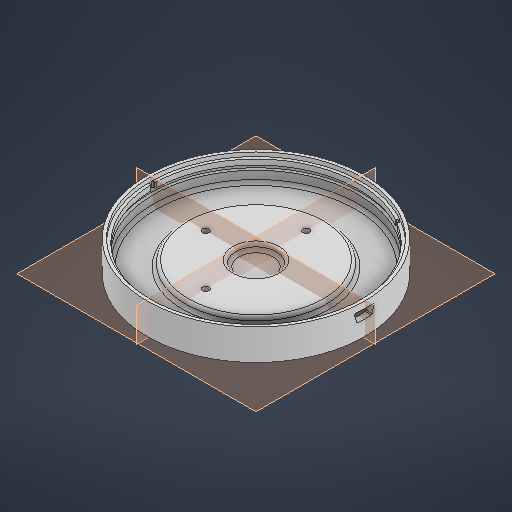
# Autodesk Inventor part: housing
Saved by Autodesk Inventor 2026 (Build 300175050, 175E)
## iProperties
Created: 2025-07-28
Part Number: housing
Material: Generic
Document SubType Name: Modeling
Designer: bruno
Density: 1 g/cm^3
Appearance: Default
Author: bruno
Autodesk Inventor part; units mm, degrees
sketch "Sketch3" plane through (0, 0, 0) normal (0, 1, 0) x (-1, 0, 0)
  circle A0 centre (0, 0) radius 54
  dimension "d4" = 108
  constraints: 1 centre point, 1 coincident
  measures "d4" diameter of A0
extrude "Extrusion2" add sketch "Sketch3" along normal blind 15.3
shell "Shell1" thickness 3 removed faces 1 at (7.7603, 15.3, 10.4365)
ref_plane "Work Plane1" through (54, 0, 0) normal (1, 0, 0) x (0, 1, 0)
sketch "Sketch5" plane through (54, 0, 0) normal (1, 0, 0) x (0, 1, 0)
  line L0 (12, 5) -> (7.5, 3.75)
  line L1 (7.5, 3.75) -> (7.5, -3.75)
  line L2 (7.5, -3.75) -> (12, -5)
  line L3 (12, -5) -> (12, 5)
  line L4 (-2.4, 0) -> (14.4, 0) projected
  line L5 (0, 7) -> (0, -7) projected
  point P0 (0, 0)
  point P1 (12, 0)
  point P2 (7.5, 0)
  dimension "d13" = 4.5
  dimension "d14" = 7.5
  dimension "d16" = 5
  dimension "d17" = 7.5
  constraints: 8 end point, 2 horizontal alignment, 2 midpoint
  measures "d13" distance between parallel lines of L3 L1
  measures "d14" distance between parallel lines of L5 L1
  measures "d16" distance from line of L4 L0.start
  measures "d17" distance of L0.end L1.end
extrude "Extrusion3" cut sketch "Sketch5" against normal blind 6
fillet "Fillet1" radius 0.5 4 edges at (52.3658, 7.5, -3.75) (52.2612, 12, -5) (52.2612, 12, 5) (52.3658, 7.5, 3.75)
sketch "Sketch6" plane through (0, 3, 0) normal (0, 1, 0) x (1, 0, 0)
  circle A0 centre (0, 0) radius 35
  circle A1 centre (0, 0) radius 10
  dimension "d19" = 70
  dimension "d22" = 20
  constraints: 2 centre point, 2 coincident
  measures "d19" diameter of A0
  measures "d22" diameter of A1
extrude "Extrusion5" add sketch "Sketch6" along normal blind 3
sketch "Sketch7" plane through (0, 0, 0) normal (0, -1, 0) x (1, 0, 0)
  circle A0 centre (0, 0) radius 35 projected
  circle A1 centre (0, 0) radius 10 projected
  circle A2 centre (0, 0) radius 54 projected
  circle A3 centre (0, 0) radius 32
  circle A4 centre (0, 0) radius 13
  dimension "d25" = 3
  dimension "d26" = 3
  constraints: 2 centre point
  measures "d25" radial gap between concentric circles of A0 A3
  measures "d26" radial gap between concentric circles of A1 A4
extrude "Extrusion6" cut sketch "Sketch7" against normal blind 3 contours A3
fillet "Fillet2" radius 2 2 edges at (-32, 3, 0) (-13, 3, 0)
fillet "Fillet3" radius 1.5 4 edges at (-35, 3, 0) (-35, 6, 0) (-10, 3, 0) (-10, 6, 0)
fillet "Fillet4" radius 1.5 1 edges at (51, 3, 0)
sketch "Sketch8" plane through (0, 0, 0) normal (1, 0, 0) x (0, 1, 0)
  line L0 (0, -32) -> (0, 32) projected
  line L1 (3, -23.4) -> (0, -23.4)
  line L2 (-1.7497, 0) -> (10.4983, 0) projected
  line L3 (0, -23.4) -> (0, -22.1)
  line L4 (0, -22.1) -> (3, -22.1)
  line L5 (3, -22.1) -> (3, -23.4)
  line L6 (4.5, 35) -> (4.5, -35) projected
  line L7 (3, -23.4) -> (3, -25)
  line L8 (0, -25) -> (8.7486, -25)
  line L9 (0, -22.1) -> (0, -21.6)
  line L10 (0, -21.6) -> (0.866, -22.1)
  point P0 (0, 0)
  dimension "d32" = 25
  dimension "d33" = 1.6
  dimension "d35" = 1.3
  dimension "d36" = 3
  dimension "d38" = 0.5
  dimension "d39" = 1
  constraints: 17 end point, 5 point on line, 2 horizontal, 1 parallel, 1 perpendicular, 1 vertical
  measures "d32" distance from line of L2 L7.end
  measures "d33" distance of L1.start L7.end
  measures "d35" distance of L1.end L3.end
  measures "d36" distance between parallel lines of L0 L5
  measures "d38" distance of L3.end L9.end
  measures "d39" distance of L9.end L10.end
revolve "Revolution1" add sketch "Sketch8" angle 360 about axis through (0, 0, -25) along (0, 1, 0) contours L0 L4 L5 L1 | L0 L10 L4
sketch "Sketch9" plane through (0, 3, -25) normal (0, -1, 0) x (1, 0, 0)
  circle A0 centre (0, 0) radius 1.6 projected
  circle A1 centre (0, 25) radius 15 projected
  circle A2 centre (0, 25) radius 30 projected
  circle A3 centre (0, 0) radius 2.9 projected
extrude "Extrusion7" cut sketch "Sketch9" against normal blind 3 contours A0
fillet "Fillet5" radius 0.5 1 edges at (0, 3, -27.9)
pattern_circular "Circular Pattern1" count 4 over 360 about axis through (0, -10, 0) along (0, 1, 0) of "Revolution1", "Extrusion7", "Fillet5" skipped copies 4
sketch "Sketch10" plane through (0, 15.3, 0) normal (0, 1, 0) x (1, 0, 0)
  circle A0 centre (0, 0) radius 51 projected
  circle A1 centre (0, 0) radius 54 projected
  circle A2 centre (0, 0) radius 52.5
  dimension "d47" = 1.5
  constraints: 1 centre point
  measures "d47" radial gap between concentric circles of A1 A2
extrude "Extrusion8" cut sketch "Sketch10" against normal blind 2 contours A2
ref_plane "Work Plane4" through (0, 8.5, 0) normal (0, 1, 0) x (-1, 0, 0)
sketch "Sketch14" plane through (0, 8.5, 0) normal (0, 1, 0) x (-1, 0, 0)
  circle A0 centre (0, 0) radius 52.5 projected
  circle A1 centre (-52.5, 0) radius 10
  line L0 (-51.5476, 9.9545) -> (0, 0)
  line L1 (0, 0) -> (-51.5476, -9.9545)
  dimension "d94" = 20
  constraints: 5 point on circle, 4 end point, 1 centre point
  measures "d94" diameter of A1
ref_plane "Work Plane5" through (0, 10.75, 0) normal (0, 1, 0) x (-1, 0, 0)
extrude "Extrusion15" cut sketch "Sketch14" along normal blind 2.25 contours A0 A1 L1 L0 | A1 L0 | L1 A1 picked at (-31.3895, 12.4879)
fillet "Fillet9" radius 1 4 edges at (50.8112, 8.5, -9.8123) (50.8112, 10.75, -9.8123) (50.8112, 8.5, 9.8123) (50.8112, 10.75, 9.8123)
sketch "Sketch18" plane through (0, 10.75, 0) normal (0, 1, 0) x (-1, 0, 0)
  arc A0 (-51.3487, -10.9346) -> (-51.3487, 10.9346) centre (0, 0) ccw projected
  circle A1 centre (52.5, -0.0002) radius 1
  circle A2 centre (0, 0) radius 11.5 projected
  line L0 (52.5, -1.0002) -> (0, 0)
  line L1 (0, 0) -> (52.4905, 0.9998)
  point P0 (-50.6191, -8.9255)
  point P1 (-50.6191, 8.9255)
  point P2 (11.4979, 0.219)
  point P3 (11.4979, -0.2191)
  point P4 (52.4905, -1)
  point P5 (-52.2934, -4.6528)
  point P6 (-52.2934, 4.6528)
  dimension "d86" = 2
  constraints: 4 end point, 4 point on circle, 1 centre point
  measures "d86" diameter of A1
extrude "Extrusion16" cut sketch "Sketch18" along normal blind 7.25 contours L0 A2 L1 A0
fillet "Fillet8" radius 0.5 4 edges at (-50.9908, 12.025, 0.9712) (-52.4905, 12.025, 0.9998) (-50.9907, 12.025, -0.9714) (-52.4905, 12.025, -1)
pattern_circular "Circular Pattern4" count 3 over 360 about axis through (0, -10, 0) along (0, 1, 0) of "Extrusion16", "Fillet8"
body "Solid2"
